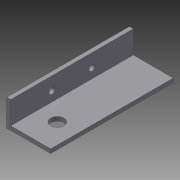
# Autodesk Inventor part: EE_Base-Rod-Rev2
Saved by Autodesk Inventor 2015 (Build 190159000, 159)
## iProperties
Created: 2016-12-24
Part Number: EE_Base-Rod-Rev2
Material: Generic
Document SubType Name: Modeling
Designer: Guy
Density: 1 g/cm^3
Appearance: Default
Mass: 13.4813 g
Surface Area: 100.129 cm^2
Volume: 13.4813 cm^3
Author: Guy
Autodesk Inventor part; units mm, degrees
ref_plane "YZ Plane" through (0, 0, 0) normal (1, 0, 0) x (0, 1, 0)
ref_plane "XZ Plane" through (0, 0, 0) normal (0, 1, 0) x (-1, 0, 0)
ref_plane "XY Plane" through (0, 0, 0) normal (0, 0, 1) x (1, 0, 0)
sketch "Sketch1" plane through (0, 0, 0) normal (0, 0, 1) x (1, 0, 0)
  line L0 (0, 0) -> (92, 0)
  line L1 (92, 0) -> (92, 20)
  line L2 (92, 20) -> (0, 20)
  line L3 (0, 20) -> (0, 0)
  dimension "d0" = 92
  dimension "d1" = 20
  constraints: 8 end point, 2 parallel, 1 horizontal, 1 perpendicular
  measures "d0" distance of L1.end L2.end
  measures "d1" distance of L2.end L0.start
extrude "Extrusion1" add sketch "Sketch1" along normal blind 3
sketch "Sketch2" plane through (0, 0, 3) normal (0, 0, 1) x (1, 0, 0)
  line L0 (0, 0) -> (92, 0) projected
  line L1 (92, 0) -> (92, 20) projected
  line L2 (92, 20) -> (0, 20) projected
  line L3 (0, 20) -> (0, 0) projected
  circle A0 centre (31, 10) radius 2.1
  circle A1 centre (61, 10) radius 2.1
  dimension "d5" = 4.2
  dimension "d6" = 31
  dimension "d7" = 10
  dimension "d8" = 10
  dimension "d9" = 31
  dimension "d10" = 4.2
  constraints: 2 centre point
  measures "d5" diameter of A0
  measures "d6" distance from line of L3 A0.centre
  measures "d7" distance from line of L2 A0.centre
  measures "d8" distance from line of L2 A1.centre
  measures "d9" distance from line of A1.centre L1
  measures "d10" diameter of A1
extrude "Extrusion2" cut sketch "Sketch2" against normal up to next contours A0 | A1
sketch "Sketch3" plane through (0, 0, 3) normal (0, 0, 1) x (1, 0, 0)
  line L0 (92, 0) -> (92, 20) projected
  line L1 (0, 0) -> (92, 0)
  line L2 (92, 0) -> (92, 3)
  line L3 (92, 3) -> (0, 3)
  line L4 (0, 3) -> (0, 0)
  dimension "d13" = 3
  constraints: 8 end point, 2 parallel, 1 horizontal, 1 perpendicular, 1 point on line
  measures "d13" distance between parallel lines of L1 L3
extrude "Extrusion3" add sketch "Sketch3" along normal blind 30
sketch "Sketch4" plane through (0, 3, 3) normal (0, 1, 0) x (1, 0, 0)
  circle A0 centre (20, -15) radius 5
  line L0 (0, 0) -> (92, 0) projected
  line L1 (0, 0) -> (0, -30) projected
  line L2 (92, -30) -> (0, -30) projected
  line L3 (92, 0) -> (92, -30) projected
  point P0 (0, 3)
  dimension "d16" = 20
  dimension "d17" = 15
  dimension "d18" = 10
  constraints: 1 centre point
  measures "d16" distance from line of L1 A0.centre
  measures "d17" distance from line of L2 A0.centre
  measures "d18" diameter of A0
extrude "Extrusion4" cut sketch "Sketch4" against normal blind 30 contours A0
body "Solid1"
